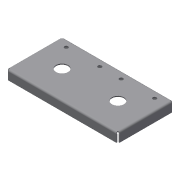
# Autodesk Inventor part: Side Plate
Saved by Autodesk Inventor 2016 (Build 200138000, 138)
## iProperties
Created: 2012-10-11
Part Number: Side Plate
Material: Generic
Document SubType Name: Sheet Metal
Designer: bruno.silveira
Density: 1 g/cm^3
Sheet Metal Rule: Default_mm
Appearance: Default
Mass: 1220.19 g
Surface Area: 5021.64 cm^2
Volume: 1220.19 cm^3
Author: bruno.silveira
Autodesk Inventor part; units mm, degrees
note: some values were not read from the file. Chosen so that the rebuilt part matches the saved one: corner form of "Plate2".
ref_plane "YZ Plane" through (0, 0, 0) normal (1, 0, 0) x (0, 1, 0)
ref_plane "XZ Plane" through (0, 0, 0) normal (0, 1, 0) x (-1, 0, 0)
ref_plane "XY Plane" through (0, 0, 0) normal (0, 0, 1) x (1, 0, 0)
sketch "Sketch1" plane through (0, 0, 0) normal (0, 0, 1) x (1, 0, 0)
  line L0 (0, 0) -> (600, 0)
  line L1 (600, 0) -> (600, 300)
  line L2 (600, 300) -> (0, 300)
  line L3 (0, 300) -> (0, 0)
  dimension "d0" = 300
  dimension "d1" = 600
  measures "d0" distance of L2.end L0.start
  measures "d1" distance of L0.start L0.end
extrude "Plate1" add sketch "Sketch1" along normal blind 5
sketch "Sketch2" plane through (595, 0, 5) normal (1, 0, 0) x (0, 1, 0)
  line L0 (300, 0) -> (0, 0)
  line L1 (0, 0) -> (0, -50)
  line L2 (0, -50) -> (300, -50)
  line L3 (300, -50) -> (300, 0)
  constraints: 6 end point, 1 horizontal, 1 perpendicular, 1 vertical
edge flange "Flange1" height 50 angle 90 thickness 5 bend radius 5 thickness toward (1, 0, 0) relief tear relief width 5 relief depth 2.5 corner gap 5 corner form 2 edges at (600, 150, 0) (0, 150, 0) (300, 0, 0) (300, 300, 0) wall of the first edge with corners at (595, 300, 5) (595, 0, 5) (595, 0, -45) (595, 300, -45)
bend "Bend1"
corner "Corner1"
sketch "Sketch3" plane through (0, 0, 5) normal (0, 0, 1) x (1, 0, 0)
  circle A0 centre (150, 150) radius 32.5
  circle A1 centre (450, 150) radius 32.5
  point P0 (0, 0)
  dimension "d13" = 65
  dimension "d14" = 65
  constraints: 2 centre point, 2 coincident, 2 other
  measures "d13" diameter of A0
  measures "d14" diameter of A1
extrude "Extrusion1" cut sketch "Sketch3" against normal blind 10
sketch "Sketch4" plane through (0, 0, 5) normal (0, 0, 1) x (1, 0, 0)
  circle A0 centre (62.5, 260) radius 10 projected
  circle A1 centre (242.5, 260) radius 10 projected
  circle A2 centre (357.5, 260) radius 10 projected
  circle A3 centre (537.5, 260) radius 10 projected
  line L0 (22.5, 236) -> (577.5, 236) projected
  line L1 (577.5, 304) -> (577.5, 236) projected
  line L2 (22.5, 304) -> (22.5, 236) projected
  line L3 (577.5, 304) -> (22.5, 304) projected
  point P0 (0, 0)
hole "Hole1" at (537.5, 260, 5) at (357.5, 260, 5) at (242.5, 260, 5) at (62.5, 260, 5) direction (0, 0, -1) diameter 20 depth 5 tip angle 118
equation "\"d22\" = Thickness"
equation "\"d3\" = BendReliefWidth"
equation "\"d4\" = BendReliefDepth"
equation "\"d5\" = MinimumRemnant"
equation "\"d6\" = BendRadius"
equation "\"d9\" = BendRadius"
equation "\"d10\" = CornerReliefSize"
equation "\"d11\" = GapSize"
equation "\"d12\" = JacobiRadiusSize"
equation "\"BendRadius\" = Thickness"
equation "\"BendReliefWidth\" = Thickness"
equation "\"BendReliefDepth\" = 0.5 * Thickness"
equation "\"TransitionRadius\" = BendRadius"
equation "\"JacobiRadiusSize\" = BendRadius"
equation "\"GapSize\" = Thickness"
equation "\"d2\" = BendRadius"
equation "\"Thickness\" = 5"
equation "\"MinimumRemnant\" = 10"
equation "\"CornerReliefSize\" = 20"
body "Solid1"
